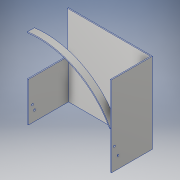
# Autodesk Inventor part: Sorter
Saved by Autodesk Inventor 2019 (Build 230136000, 136)
## iProperties
Created: 2018-11-20
Part Number: Sorter
Material: Aluminum 6061
Document SubType Name: Modeling
Designer: User
Density: 2.7 g/cm^3
Appearance: Aluminum - Flat
Author: User
Autodesk Inventor part; units mm, degrees
ref_plane "YZ Plane" through (0, 0, 0) normal (1, 0, 0) x (0, 1, 0)
ref_plane "XZ Plane" through (0, 0, 0) normal (0, 1, 0) x (-1, 0, 0)
ref_plane "XY Plane" through (0, 0, 0) normal (0, 0, 1) x (1, 0, 0)
sketch "Sketch1" plane through (0, 0, 0) normal (0, 0, 1) x (1, 0, 0)
  line L0 (0, 0) -> (156.1084, 0)
  line L1 (156.1084, 0) -> (156.1084, 149.7584)
  line L2 (156.1084, 149.7584) -> (0, 149.7584)
  line L3 (0, 149.7584) -> (0, 0)
  dimension "d0" = 156.1084
  dimension "d1" = 149.7584
  constraints: 8 end point, 2 parallel, 1 horizontal, 1 perpendicular
  measures "d0" distance of L2.end L1.end
  measures "d1" distance between parallel lines of L2 L0
extrude "Extrusion1" add sketch "Sketch1" along normal blind 76.2
sketch "Sketch2" plane through (0, 0, 0) normal (0, -1, 0) x (1, 0, 0)
  line L0 (156.1084, 0) -> (156.1084, 76.2) projected
  line L1 (0, 0) -> (156.1084, 0) projected
  line L2 (0, 76.2) -> (156.1084, 76.2) projected
  line L3 (154.2542, 1.8542) -> (1.8542, 1.8542)
  line L4 (1.8542, 1.8542) -> (1.8542, 76.2)
  line L5 (1.8542, 76.2) -> (154.2542, 76.2)
  line L6 (154.2542, 76.2) -> (154.2542, 1.8542)
  dimension "d4" = 1.8542
  dimension "d5" = 1.8542
  dimension "d6" = 152.4
  dimension "d49" = 156.1084
  constraints: 8 end point, 2 parallel, 1 horizontal, 1 perpendicular, 1 point on line
  measures "d4" distance from line of L0 L3.start
  measures "d5" distance from line of L1 L3.start
  measures "d6" distance of L4.end L5.end
  measures "d49" distance of L1.start L0.start
extrude "Extrusion2" cut sketch "Sketch2" against normal blind 228.6
sketch "Sketch3" plane through (0, 0, 76.2) normal (0, 0, 1) x (1, 0, 0)
  line L0 (1.8542, 0) -> (1.8542, 149.7584) projected
  line L1 (0, 149.7584) -> (1.8542, 149.7584)
  line L2 (1.8542, 149.7584) -> (1.8542, 73.5584)
  line L3 (1.8542, 73.5584) -> (0, 73.5584)
  line L4 (0, 73.5584) -> (0, 149.7584)
  line L5 (1.8542, 149.7584) -> (154.2542, 149.7584) projected
  point P0 (0, 0)
  dimension "d9" = 76.2
  constraints: 8 end point, 2 parallel, 2 point on line, 1 horizontal, 1 perpendicular
  measures "d9" distance of L1.end L2.end
extrude "Extrusion3" cut sketch "Sketch3" against normal blind 74.3458
sketch "Sketch9" plane through (0, 0, 76.2) normal (0, 0, 1) x (1, 0, 0)
  line L0 (154.2542, 149.7584) -> (154.2542, 0) projected
  line L1 (0, 73.5584) -> (0, 149.7584) projected
  arc A0 (154.2542, 69.7484) -> (0, 149.3143) centre (20.8699, 0.4656) ccw
  line L2 (0, 149.3143) -> (218.1484, 149.3143) construction
  line L3 (154.2542, 69.7484) -> (152.4, 69.7484)
  arc A1 (152.4, 69.7484) -> (0, 147.4601) centre (20.5853, -0.4615) ccw
  line L4 (156.1084, 149.7584) -> (154.2542, 149.7584) projected
  line L5 (0, 149.3143) -> (0, 147.4601)
  point P0 (0, 0)
  dimension "d23" = 1.8542
  dimension "d24" = 1.8542
  dimension "d50" = 0.9271
  dimension "d51" = 80.01
  constraints: 6 end point, 4 point on circle, 2 centre point, 2 horizontal, 2 point on line, 1 vertical
  measures "d23" distance of L3.start L3.end
  measures "d24" distance of L2.start L5.end
  measures "d50" vertical distance of A0.centre A1.centre
  measures "d51" distance between parallel lines of L3 L4
extrude "Extrusion7" add sketch "Sketch9" against normal blind 12.7
sketch "Sketch10" plane through (0, 0, 0) normal (-1, 0, 0) x (0, 0, 1)
  line L0 (0, 0) -> (76.2, 0) projected
  line L1 (76.2, 149.7584) -> (76.2, 0) projected
  point P0 (64.9986, 18.5674)
  point P1 (76.2, 73.5584)
  point P2 (68.8594, 29.21)
  dimension "d27" = 18.5674
  dimension "d28" = 11.2014
  dimension "d29" = 7.3406
  dimension "d30" = 29.21
  measures "d27" distance from line of L0 point (64.999, 18.567)
  measures "d28" distance from line of L1 point (64.999, 18.567)
  measures "d29" distance from line of L1 point (68.859, 29.21)
  measures "d30" distance from line of L0 point (68.859, 29.21)
hole "Hole1" at (0, 29.21, 68.8594) at (0, 18.5674, 64.9986) direction (1, 0, 0) diameter 3.7084 depth 1.8542
sketch "Sketch11" plane through (156.1084, 0, 0) normal (1, 0, 0) x (0, 0, -1)
  line L0 (0, 0) -> (-76.2, 0) projected
  line L1 (-76.2, 0) -> (-76.2, 149.7584) projected
  point P0 (-70.7898, 40.1574)
  point P1 (-64.0842, 21.7678)
  dimension "d38" = 40.1574
  dimension "d39" = 5.4102
  dimension "d40" = 12.1158
  dimension "d41" = 21.7678
  measures "d38" distance from line of L0 point (-70.79, 40.157)
  measures "d39" distance from line of L1 point (-70.79, 40.157)
  measures "d40" distance from line of L1 point (-64.084, 21.768)
  measures "d41" distance from line of L0 point (-64.084, 21.768)
hole "Hole2" at (156.1084, 40.1574, 70.7898) at (156.1084, 21.7678, 64.0842) direction (-1, 0, 0) diameter 3.7084 depth 1.8542
equation "\"d6\" = d49 - 2 * d5"
body "Solid1"
